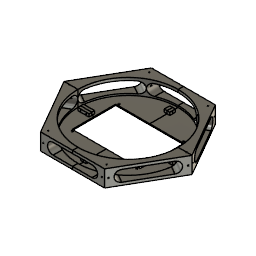
BoTech.StarClock.Top (Autodesk Fusion 360 design; units mm, degrees)
Autodesk Fusion 360 part; units mm, degrees
note: some values were not read from the file. Chosen so that the rebuilt part matches the saved one: which bodies a step acts on. Set by a fixed rule: which sketch regions a step uses.
sketch "Skizze1" plane through (0, 0, 0) normal (0, 0, 1) x (1, 0, 0)
  line L0 (-61, 39) -> (61, 39)
  line L1 (61, 39) -> (61, -39)
  line L2 (61, -39) -> (-61, -39)
  line L3 (-61, -39) -> (-61, 39)
  line L4 (0, 0) -> (0, 39)
  line L5 (61, 44.5) -> (61, -44.5)
  line L6 (61, -39) -> (55, -39)
  line L7 (55, -39) -> (55, -44.5)
  line L8 (55, -44.5) -> (61, -44.5)
  line L9 (61, -44.5) -> (61, -39)
  line L10 (-61, -39) -> (-55, -39)
  line L11 (-55, -39) -> (-55, -44.5)
  line L12 (-55, -44.5) -> (-61, -44.5)
  line L13 (-61, -44.5) -> (-61, -39)
  line L14 (-61, 39) -> (-55, 39)
  line L15 (-55, 39) -> (-55, 44.5)
  line L16 (-55, 44.5) -> (-61, 44.5)
  line L17 (-61, 44.5) -> (-61, 39)
  line L18 (61, 39) -> (55, 39)
  line L19 (55, 39) -> (55, 44.5)
  line L20 (55, 44.5) -> (61, 44.5)
  line L21 (61, 44.5) -> (61, 39)
  circle A0 centre (58, 42) radius 1.5
  circle A1 centre (-58, 42) radius 1.5
  circle A2 centre (-58, -42) radius 1.5
  line L22 (58, 42) -> (58, -42)
  circle A3 centre (58, -42) radius 1.5
  line L23 (-70, 50) -> (70, 50)
  line L24 (70, 50) -> (70, -50)
  line L25 (70, -50) -> (-70, -50)
  line L26 (-70, -50) -> (-70, 50)
  line L27 (115, 0) -> (57.5, 99.5929)
  line L28 (57.5, 99.5929) -> (-57.5, 99.5929)
  line L29 (-57.5, 99.5929) -> (-115, 0)
  line L30 (-115, 0) -> (-57.5, -99.5929)
  line L31 (-57.5, -99.5929) -> (57.5, -99.5929)
  line L32 (57.5, -99.5929) -> (115, 0)
  circle A4 centre (0, 0) radius 90
  line L33 (-57.5, 99.5929) -> (57.5, -99.5929)
  line L34 (57.5, 99.5929) -> (-57.5, -99.5929)
  line L35 (-115, 0) -> (115, 0)
  circle A5 centre (-105, 0) radius 1
  line L36 (-57.5, 99.5929) -> (-52.5, 90.9327)
  circle A6 centre (-52.5, 90.9327) radius 1
  line L37 (57.5, 99.5929) -> (52.5, 90.9327)
  circle A7 centre (52.5, 90.9327) radius 1
  line L38 (115, 0) -> (105, 0)
  circle A8 centre (105, 0) radius 1
  line L39 (57.5, -99.5929) -> (52.5, -90.9327)
  circle A9 centre (52.5, -90.9327) radius 1
  line L40 (-57.5, -99.5929) -> (-52.5, -90.9327)
  circle A10 centre (-52.5, -90.9327) radius 1
  line L41 (-0.0002, 220) -> (-190.5257, 109.9998)
  line L42 (-190.5257, 109.9998) -> (-190.5255, -110.0002)
  line L43 (-190.5255, -110.0002) -> (0.0002, -220)
  line L44 (0.0002, -220) -> (190.5257, -109.9998)
  line L45 (190.5257, -109.9998) -> (190.5255, 110.0002)
  line L46 (190.5255, 110.0002) -> (-0.0002, 220)
  line L47 (-0.0002, 220) -> (-57.5, 99.5929)
  line L48 (-0.0002, 220) -> (57.5, 99.5929)
  line L49 (57.5, 99.5929) -> (190.5255, 110.0002)
  line L50 (190.5255, 110.0002) -> (127.0171, 0.0001)
  line L51 (127.0171, 0.0001) -> (190.5257, -109.9998)
  line L52 (57.5, -99.5929) -> (190.5257, -109.9998)
  line L53 (57.5, -99.5929) -> (0.0002, -220)
  line L54 (-57.5, -99.5929) -> (0.0002, -220)
  line L55 (-57.5, -99.5929) -> (-190.5255, -110.0002)
  line L56 (-190.5255, -110.0002) -> (-115, 0)
  line L57 (-115, 0) -> (-190.5257, 109.9998)
  line L58 (-57.5, 99.5929) -> (-190.5257, 109.9998)
  line L59 (57.5, 99.5929) -> (0, 99.5929)
  dimension "d1" = 122
  dimension "d2" = 78
  dimension "d3" = 39
  dimension "d4" = 89
  dimension "d5" = 6
  dimension "d7" = 5.5
  dimension "d8" = 6
  dimension "d9" = 5.5
  dimension "d10" = 6
  dimension "d11" = 5.5
  dimension "d12" = 6
  dimension "d13" = 5.5
  dimension "d14" = 3
  dimension "d17" = 3
  dimension "d19" = 3
  dimension "d22" = 84
  dimension "d23" = 3
  dimension "d24" = 140
  dimension "d25" = 100
  dimension "d26" = 115
  dimension "d27" = 180
  dimension "d28" = 2
  dimension "d29" = 10
  dimension "d30" = 2
  dimension "d31" = 10
  dimension "d32" = 2
  dimension "d33" = 10
  dimension "d34" = 2
  dimension "d35" = 10
  dimension "d36" = 2
  dimension "d37" = 10
  dimension "d38" = 2
  dimension "d43" = 220
  dimension "d44" = 57.5
  constraint horizontal L0
  constraint vertical L1
  constraint horizontal L2
  constraint vertical L3
  constraint coincident L4.start A4.centre
  constraint perpendicular L2 L4
  constraint perpendicular L2 L5
  constraint coincident L2 L6.end
  constraint vertical L7
  constraint horizontal L8
  constraint vertical L9
  constraint horizontal L10
  constraint vertical L11
  constraint horizontal L12
  constraint vertical L13
  constraint horizontal L14
  constraint vertical L15
  constraint horizontal L16
  constraint vertical L17
  constraint horizontal L18
  constraint vertical L19
  constraint horizontal L20
  constraint vertical L21
  constraint perpendicular L0 L22
  constraint coincident A0.centre L22.start
  constraint coincident L22.end A3.centre
  constraint horizontal L23
  constraint vertical L24
  constraint horizontal L25
  constraint vertical L26
  constraint horizontal L35
  constraint coincident L35 A5.centre
  constraint coincident L33 L36.end
  constraint coincident L36.end A6.centre
  constraint coincident L34 L37.end
  constraint coincident L37.end A7.centre
  constraint coincident L35 L38.end
  constraint coincident L38.end A8.centre
  constraint coincident L33 L39.end
  constraint coincident L39.end A9.centre
  constraint coincident L34 L40.end
  constraint coincident L40.end A10.centre
  constraint perpendicular L46 L50
  constraint perpendicular L44 L51
  constraint parallel L28 L59
  measures "d1" distance of L0.start L0.end
  measures "d2" distance of L0.start L2.end
  measures "d3" distance of L4.start L4.end
  measures "d4" distance of L5.start L5.end
  measures "d5" distance of L1.end L6.end
  measures "d7" distance of L1.end L5.end
  measures "d8" distance of L2.end L10.end
  measures "d9" distance of L2.end L12.end
  measures "d10" distance of L0.start L14.end
  measures "d11" distance of L0.start L16.end
  measures "d12" distance of L0.end L18.end
  measures "d13" distance of L0.end L5.start
  measures "d14" diameter of A0
  measures "d17" diameter of A1
  measures "d19" diameter of A2
  measures "d22" distance of A0.centre L22.end
  measures "d23" diameter of A3
  measures "d24" distance of L23.start L23.end
  measures "d25" distance of L23.start L25.end
  measures "d26" distance of L27.start L4.start
  measures "d27" diameter of A4
  measures "d28" diameter of A5
  measures "d29" distance of L28.end L36.end
  measures "d30" diameter of A6
  measures "d31" distance of L27.end L37.end L4.start
  measures "d32" diameter of A7 L4.start
  measures "d33" distance of L27.start L38.end
  measures "d34" diameter of A8
  measures "d35" distance of L31.end L39.end
  measures "d36" diameter of A9
  measures "d37" distance of L30.end L40.end
  measures "d38" diameter of A10
  measures "d43" distance of L41.start L4.start
  measures "d44" distance of L27.end L59.end L4.start
extrude "Extrusion1" add sketch "Skizze1" along normal blind 30 contours L29 A4 L33 L35 A5 L36 A6 | L30 A4 L34 L35 A5 L40 A10 | L28 A4 L33 L34 L36 A6 L37 A7 L59 | L31 A4 L33 L34 L39 A9 L40 A10 | L27 A4 L34 L35 L37 A7 L38 A8 | L32 A4 L33 L35 L38 A8 L39 A9 makes body 1
extrude "Extrusion2" add sketch "Skizze1" along normal blind 2 contours L0 L14 L15 L16 L17 | L0 L3 L15 L16 L17 L23 L26 L33 L35 | L2 L3 L11 L12 L13 L25 L26 L34 L35 | L0 L23 L33 L34 | L2 L10 L11 L12 L13 | L23 L26 A4 L33 L35 | L25 L26 A4 L34 L35 | L23 A4 L33 L34 | L2 L25 L33 L34 | L1 L2 L5 L7 L8 L9 L24 L25 L33 L35 | L0 L1 L5 L19 L20 L21 L23 L24 L34 L35 | L23 L24 A4 L34 L35 | L25 A4 L33 L34 | L35 A5 | L35 A5 | L2 L5 L6 L7 L8 L9 | L24 L25 A4 L33 L35 | L0 L5 L18 L19 L20 L21 | L33 L36 A6 | L33 L36 A6 | L34 L40 A10 | L34 L40 A10 | L34 L37 A7 | L34 L37 A7 | L33 L39 A9 | L33 L39 A9 | L35 L38 A8 | L35 L38 A8 bodies 1
sketch "Skizze2" plane through (0, -99.5929, 0) normal (0, -1, 0) x (1, 0, 0)
  line L0 (-57.5, 0) -> (57.5, 0)
  line L1 (57.5, 0) -> (57.5, 30)
  line L2 (57.5, 30) -> (-57.5, 30)
  line L3 (-57.5, 30) -> (-57.5, 0)
  line L4 (57.5, 30) -> (57.5, 0)
  line L5 (-57.5, 30) -> (57.5, 30)
  circle A0 centre (-52.5, 15) radius 2.5
  circle A1 centre (52.5, 15) radius 3.5
  circle A2 centre (-52.5, 15) radius 3.5
  line L6 (-57.5, 0) -> (-57.5, 30)
  circle A3 centre (52.5, 15) radius 1
  line L7 (47.5, 0) -> (47.5, 30)
  circle A4 centre (-52.5, 15) radius 1
  line L8 (57.5, 0) -> (-57.5, 0)
  line L9 (-47.5, 30) -> (-47.5, 0)
  circle A5 centre (52.5, 15) radius 2.5
  line L10 (-35, 25) -> (35, 25)
  line L11 (35, 25) -> (35, 5)
  line L12 (35, 5) -> (-35, 5)
  arc A6 (-35, 25) -> (-35, 5) centre (-35, 15) ccw
  arc A7 (35, 5) -> (35, 25) centre (35, 15) ccw
  point P0 (-57.5, 15)
  dimension "d45" = 115
  dimension "d46" = 30
  dimension "d47" = 2
  dimension "d48" = 5
  dimension "d49" = 2
  dimension "d50" = 5
  constraint horizontal L8
  constraint vertical L6
  constraint horizontal L5
  constraint vertical L4
  constraint concentric A3 A5
  constraint concentric A0 A4
  constraint coincident L9.start L5
  constraint coincident L9.end L8
  constraint perpendicular L8 L9
  constraint coincident L7.start L8
  constraint coincident L7.end L5
  constraint perpendicular L5 L7
  constraint concentric A0 A2
  constraint concentric A1 A3
  constraint parallel L5 L10
  constraint perpendicular L8 L11
  constraint perpendicular L11 L12
  constraint tangent L10 A6
  constraint tangent L12 A7
  measures "d45" distance of L0.end L0.start
  measures "d46" distance of L0.end L1.end
  measures "d47" diameter of A3
  measures "d48" diameter of A5
  measures "d49" diameter of A4
  measures "d50" diameter of A0
sketch "Skizze3" plane through (86.25, -49.7965, 0) normal (0.866025, -0.5, 0) x (0.5, 0.866025, 0)
  line L0 (-57.5, 0) -> (57.5, 0)
  line L1 (57.5, 0) -> (57.5, 30)
  line L2 (57.5, 30) -> (-57.5, 30)
  line L3 (-57.5, 30) -> (-57.5, 0)
  line L4 (35, 5) -> (-35, 5)
  arc A0 (-35, 25) -> (-35, 5) centre (-35, 15) ccw
  circle A1 centre (-52.5, 15) radius 3.5
  circle A2 centre (52.5, 15) radius 1
  line L5 (57.5, 30) -> (57.5, 0)
  line L6 (35, 25) -> (35, 5)
  line L7 (-47.5, 30) -> (-47.5, 0)
  circle A3 centre (52.5, 15) radius 2.5
  line L8 (57.5, 0) -> (57.5, 30)
  circle A4 centre (-52.5, 15) radius 2.5
  line L9 (-57.5, 0) -> (57.5, 0)
  circle A5 centre (52.5, 15) radius 3.5
  arc A6 (35, 5) -> (35, 25) centre (35, 15) ccw
  line L10 (57.5, 0) -> (-57.5, 0)
  line L11 (-57.5, 30) -> (57.5, 30)
  line L12 (-57.5, 0) -> (-57.5, 30)
  circle A7 centre (-52.5, 15) radius 1
  line L13 (-35, 25) -> (35, 25)
  line L14 (-57.5, 30) -> (-57.5, 0)
  line L15 (47.5, 0) -> (47.5, 30)
  line L16 (57.5, 30) -> (-57.5, 30)
  point P0 (-57.5, 15)
  dimension "d53" = 115
  dimension "d54" = 30
  dimension "d55" = 2
  dimension "d56" = 5
  dimension "d57" = 2
  dimension "d58" = 5
  constraint horizontal L10
  constraint vertical L12
  constraint horizontal L11
  constraint vertical L5
  constraint concentric A2 A3
  constraint concentric A4 A7
  constraint coincident L7.start L11
  constraint coincident L7.end L10
  constraint perpendicular L7 L10
  constraint coincident L15.start L10
  constraint coincident L15.end L11
  constraint perpendicular L11 L15
  constraint concentric A1 A4
  constraint concentric A2 A5
  constraint parallel L11 L13
  constraint perpendicular L6 L10
  constraint perpendicular L4 L6
  constraint tangent A0 L13
  constraint tangent L4 A6
  measures "d53" distance of L0.start L0.end
  measures "d54" distance of L1.end L0.end
  measures "d55" diameter of A2
  measures "d56" diameter of A3
  measures "d57" diameter of A7
  measures "d58" diameter of A4
sketch "Skizze4" plane through (86.25, 49.7965, 0) normal (0.866025, 0.5, 0) x (-0.5, 0.866025, 0)
  line L0 (-57.5, 0) -> (57.5, 0)
  line L1 (57.5, 0) -> (57.5, 30)
  line L2 (57.5, 30) -> (-57.5, 30)
  line L3 (-57.5, 30) -> (-57.5, 0)
  line L4 (35, 5) -> (-35, 5)
  arc A0 (-35, 25) -> (-35, 5) centre (-35, 15) ccw
  circle A1 centre (-52.5, 15) radius 3.5
  circle A2 centre (52.5, 15) radius 1
  line L5 (57.5, 30) -> (57.5, 0)
  line L6 (35, 25) -> (35, 5)
  line L7 (-47.5, 30) -> (-47.5, 0)
  circle A3 centre (52.5, 15) radius 2.5
  line L8 (57.5, 0) -> (57.5, 30)
  circle A4 centre (-52.5, 15) radius 2.5
  line L9 (-57.5, 0) -> (57.5, 0)
  circle A5 centre (52.5, 15) radius 3.5
  arc A6 (35, 5) -> (35, 25) centre (35, 15) ccw
  line L10 (57.5, 0) -> (-57.5, 0)
  line L11 (-57.5, 30) -> (57.5, 30)
  line L12 (-57.5, 0) -> (-57.5, 30)
  circle A7 centre (-52.5, 15) radius 1
  line L13 (-35, 25) -> (35, 25)
  line L14 (-57.5, 30) -> (-57.5, 0)
  line L15 (47.5, 0) -> (47.5, 30)
  line L16 (57.5, 30) -> (-57.5, 30)
  point P0 (-57.5, 15)
  dimension "d59" = 115
  dimension "d60" = 30
  dimension "d61" = 2
  dimension "d62" = 5
  dimension "d63" = 2
  dimension "d64" = 5
  constraint horizontal L10
  constraint vertical L12
  constraint horizontal L11
  constraint vertical L5
  constraint concentric A2 A3
  constraint concentric A4 A7
  constraint coincident L7.start L11
  constraint coincident L7.end L10
  constraint perpendicular L7 L10
  constraint coincident L15.start L10
  constraint coincident L15.end L11
  constraint perpendicular L11 L15
  constraint concentric A1 A4
  constraint concentric A2 A5
  constraint parallel L11 L13
  constraint perpendicular L6 L10
  constraint perpendicular L4 L6
  constraint tangent A0 L13
  constraint tangent L4 A6
  measures "d59" distance of L0.start L0.end
  measures "d60" distance of L1.end L0.end
  measures "d61" diameter of A2
  measures "d62" diameter of A3
  measures "d63" diameter of A7
  measures "d64" diameter of A4
sketch "Skizze5" plane through (0, 99.5929, 0) normal (0, 1, 0) x (-1, 0, 0)
  line L0 (-57.5, 0) -> (57.5, 0)
  line L1 (57.5, 0) -> (57.5, 30)
  line L2 (57.5, 30) -> (-57.5, 30)
  line L3 (-57.5, 30) -> (-57.5, 0)
  line L4 (35, 5) -> (-35, 5)
  arc A0 (-35, 25) -> (-35, 5) centre (-35, 15) ccw
  circle A1 centre (-52.5, 15) radius 3.5
  circle A2 centre (52.5, 15) radius 1
  line L5 (57.5, 30) -> (57.5, 0)
  line L6 (35, 25) -> (35, 5)
  line L7 (-47.5, 30) -> (-47.5, 0)
  circle A3 centre (52.5, 15) radius 2.5
  line L8 (57.5, 0) -> (57.5, 30)
  circle A4 centre (-52.5, 15) radius 2.5
  line L9 (-57.5, 0) -> (57.5, 0)
  circle A5 centre (52.5, 15) radius 3.5
  arc A6 (35, 5) -> (35, 25) centre (35, 15) ccw
  line L10 (57.5, 0) -> (-57.5, 0)
  line L11 (-57.5, 30) -> (57.5, 30)
  line L12 (-57.5, 0) -> (-57.5, 30)
  circle A7 centre (-52.5, 15) radius 1
  line L13 (-35, 25) -> (35, 25)
  line L14 (-57.5, 30) -> (-57.5, 0)
  line L15 (47.5, 0) -> (47.5, 30)
  line L16 (57.5, 30) -> (-57.5, 30)
  point P0 (-57.5, 15)
  dimension "d65" = 115
  dimension "d66" = 30
  dimension "d67" = 2
  dimension "d68" = 5
  dimension "d69" = 2
  dimension "d70" = 5
  constraint horizontal L10
  constraint vertical L12
  constraint horizontal L11
  constraint vertical L5
  constraint concentric A2 A3
  constraint concentric A4 A7
  constraint coincident L7.start L11
  constraint coincident L7.end L10
  constraint perpendicular L7 L10
  constraint coincident L15.start L10
  constraint coincident L15.end L11
  constraint perpendicular L11 L15
  constraint concentric A1 A4
  constraint concentric A2 A5
  constraint parallel L11 L13
  constraint perpendicular L6 L10
  constraint perpendicular L4 L6
  constraint tangent A0 L13
  constraint tangent L4 A6
  measures "d65" distance of L0.start L0.end
  measures "d66" distance of L1.end L0.end
  measures "d67" diameter of A2
  measures "d68" diameter of A3
  measures "d69" diameter of A7
  measures "d70" diameter of A4
sketch "Skizze6" plane through (-86.25, 49.7965, 0) normal (-0.866025, 0.5, 0) x (-0.5, -0.866025, 0)
  line L0 (-57.5, 0) -> (57.5, 0)
  line L1 (57.5, 0) -> (57.5, 30)
  line L2 (57.5, 30) -> (-57.5, 30)
  line L3 (-57.5, 30) -> (-57.5, 0)
  line L4 (35, 5) -> (-35, 5)
  arc A0 (-35, 25) -> (-35, 5) centre (-35, 15) ccw
  circle A1 centre (-52.5, 15) radius 3.5
  circle A2 centre (52.5, 15) radius 1
  line L5 (57.5, 30) -> (57.5, 0)
  line L6 (35, 25) -> (35, 5)
  line L7 (-47.5, 30) -> (-47.5, 0)
  circle A3 centre (52.5, 15) radius 2.5
  line L8 (57.5, 0) -> (57.5, 30)
  circle A4 centre (-52.5, 15) radius 2.5
  line L9 (-57.5, 0) -> (57.5, 0)
  circle A5 centre (52.5, 15) radius 3.5
  arc A6 (35, 5) -> (35, 25) centre (35, 15) ccw
  line L10 (57.5, 0) -> (-57.5, 0)
  line L11 (-57.5, 30) -> (57.5, 30)
  line L12 (-57.5, 0) -> (-57.5, 30)
  circle A7 centre (-52.5, 15) radius 1
  line L13 (-35, 25) -> (35, 25)
  line L14 (-57.5, 30) -> (-57.5, 0)
  line L15 (47.5, 0) -> (47.5, 30)
  line L16 (57.5, 30) -> (-57.5, 30)
  point P0 (-57.5, 15)
  dimension "d71" = 115
  dimension "d72" = 30
  dimension "d73" = 2
  dimension "d74" = 5
  dimension "d75" = 2
  dimension "d76" = 5
  constraint horizontal L10
  constraint vertical L12
  constraint horizontal L11
  constraint vertical L5
  constraint concentric A2 A3
  constraint concentric A4 A7
  constraint coincident L7.start L11
  constraint coincident L7.end L10
  constraint perpendicular L7 L10
  constraint coincident L15.start L10
  constraint coincident L15.end L11
  constraint perpendicular L11 L15
  constraint concentric A1 A4
  constraint concentric A2 A5
  constraint parallel L11 L13
  constraint perpendicular L6 L10
  constraint perpendicular L4 L6
  constraint tangent A0 L13
  constraint tangent L4 A6
  measures "d71" distance of L0.start L0.end
  measures "d72" distance of L1.end L0.end
  measures "d73" diameter of A2
  measures "d74" diameter of A3
  measures "d75" diameter of A7
  measures "d76" diameter of A4
sketch "Skizze7" plane through (-86.25, -49.7965, 0) normal (-0.866025, -0.5, 0) x (0.5, -0.866025, 0)
  line L0 (-57.5, 0) -> (57.5, 0)
  line L1 (57.5, 0) -> (57.5, 30)
  line L2 (57.5, 30) -> (-57.5, 30)
  line L3 (-57.5, 30) -> (-57.5, 0)
  line L4 (35, 5) -> (-35, 5)
  arc A0 (-35, 25) -> (-35, 5) centre (-35, 15) ccw
  circle A1 centre (-52.5, 15) radius 3.5
  circle A2 centre (52.5, 15) radius 1
  line L5 (57.5, 30) -> (57.5, 0)
  line L6 (35, 25) -> (35, 5)
  line L7 (-47.5, 30) -> (-47.5, 0)
  circle A3 centre (52.5, 15) radius 2.5
  line L8 (57.5, 0) -> (57.5, 30)
  circle A4 centre (-52.5, 15) radius 2.5
  line L9 (-57.5, 0) -> (57.5, 0)
  circle A5 centre (52.5, 15) radius 3.5
  arc A6 (35, 5) -> (35, 25) centre (35, 15) ccw
  line L10 (57.5, 0) -> (-57.5, 0)
  line L11 (-57.5, 30) -> (57.5, 30)
  line L12 (-57.5, 0) -> (-57.5, 30)
  circle A7 centre (-52.5, 15) radius 1
  line L13 (-35, 25) -> (35, 25)
  line L14 (-57.5, 30) -> (-57.5, 0)
  line L15 (47.5, 0) -> (47.5, 30)
  line L16 (57.5, 30) -> (-57.5, 30)
  point P0 (-57.5, 15)
  dimension "d77" = 115
  dimension "d78" = 30
  dimension "d79" = 2
  dimension "d80" = 5
  dimension "d81" = 2
  dimension "d82" = 5
  constraint horizontal L10
  constraint vertical L12
  constraint horizontal L11
  constraint vertical L5
  constraint concentric A2 A3
  constraint concentric A4 A7
  constraint coincident L7.start L11
  constraint coincident L7.end L10
  constraint perpendicular L7 L10
  constraint coincident L15.start L10
  constraint coincident L15.end L11
  constraint perpendicular L11 L15
  constraint concentric A1 A4
  constraint concentric A2 A5
  constraint parallel L11 L13
  constraint perpendicular L6 L10
  constraint perpendicular L4 L6
  constraint tangent A0 L13
  constraint tangent L4 A6
  measures "d77" distance of L0.start L0.end
  measures "d78" distance of L1.end L0.end
  measures "d79" diameter of A2
  measures "d80" diameter of A3
  measures "d81" diameter of A7
  measures "d82" diameter of A4
extrude "Extrusion3" cut sketch "Skizze2" against normal blind 28 contours A3 | A4 | L10 L11 L12 A6 | L11 A7 bodies 1
extrude "Extrusion4" cut sketch "Skizze3" against normal blind 28 contours L4 A0 L6 L13 | L6 A6 | A2 | A7 bodies 1
extrude "Extrusion5" cut sketch "Skizze4" against normal blind 28 contours L4 A0 L6 L13 | L6 A6 | A2 | A7 bodies 1
extrude "Extrusion6" cut sketch "Skizze5" against normal blind 28 contours L4 A0 L6 L13 | L6 A6 | A2 | A7 bodies 1
extrude "Extrusion7" cut sketch "Skizze6" against normal blind 28 contours L4 A0 L6 L13 | L6 A6 | A2 | A7 bodies 1
extrude "Extrusion8" cut sketch "Skizze7" against normal blind 28 contours L4 A0 L6 L13 | L6 A6 | A2 | A7 bodies 1
sketch "Skizze8" plane through (0, 0, 2) normal (0, 0, 1) x (-1, 0, 0)
  circle A0 centre (-58, -42) radius 1.5
  circle A1 centre (-58, 42) radius 1.5
  line L0 (-61, -39) -> (-61, 39)
  line L1 (-61, 39) -> (61, 39)
  line L2 (61, 39) -> (61, -39)
  line L3 (61, -39) -> (-61, -39)
  circle A2 centre (58, 42) radius 1.5
  circle A3 centre (58, -42) radius 1.5
  circle A4 centre (0, 0) radius 90
  line L4 (65, 5) -> (85, 5)
  line L5 (85, 5) -> (85, -5)
  line L6 (85, -5) -> (65, -5)
  line L7 (65, -5) -> (65, 5)
  line L8 (0, -20) -> (0, 10)
  line L9 (-85, -5) -> (-65, -5)
  line L10 (-65, -5) -> (-65, 5)
  line L11 (-85, 5) -> (-85, -5)
  line L12 (-65, 5) -> (-85, 5)
  line L13 (5, 80) -> (-5, 80)
  line L14 (-5, 80) -> (-5, 70)
  line L15 (-5, 70) -> (5, 70)
  line L16 (5, 70) -> (5, 80)
  line L17 (15, 0) -> (-20, 0)
  line L18 (5, -80) -> (-5, -80)
  line L19 (-5, -80) -> (-5, -70)
  line L20 (5, -70) -> (5, -80)
  line L21 (-5, -70) -> (5, -70)
  dimension "d101" = 10
  dimension "d102" = 10
  constraint horizontal L4
  constraint vertical L5
  constraint horizontal L6
  constraint vertical L7
  constraint vertical L8
  constraint symmetric L4.start L8 L10.end
  constraint symmetric L4.end L8 L11.start
  constraint symmetric L5.end L8 L9.start
  constraint symmetric L6.end L8 L9.end
  constraint horizontal L13
  constraint vertical L14
  constraint horizontal L15
  constraint vertical L16
  constraint perpendicular L8 L17
  constraint symmetric L13.start L17 L18.start
  constraint symmetric L13.end L17 L18.end
  constraint symmetric L14.end L17 L19.end
  constraint symmetric L15.end L17 L20.start
  measures "d101" distance of L13.start L13.end
  measures "d102" distance of L13.start L15.end
extrude "Extrusion9" add sketch "Skizze8" along normal blind 5 contours L4 L5 L6 L7 | L9 L10 L11 L12 | L13 L14 L15 L16 | L18 L19 L20 L21 bodies 1
sketch "Skizze9" plane through (0, -5, 0) normal (0, -1, 0) x (1, 0, 0)
  line L0 (-85, 2) -> (-65, 2)
  line L1 (-65, 2) -> (-65, 7)
  line L2 (-65, 7) -> (-85, 7)
  line L3 (-85, 7) -> (-85, 2)
  line L4 (-85, 7) -> (-65, 7)
  line L5 (-65, 7) -> (-65, 2)
  line L6 (-65, 2) -> (-85, 2)
  line L7 (-85, 2) -> (-85, 7)
  line L8 (-85, 4.5) -> (-80, 4.5)
  circle A0 centre (-80, 4.5) radius 1
  line L9 (-65, 4.5) -> (-70, 4.5)
  circle A1 centre (-70, 4.5) radius 1
  line L10 (0, 0) -> (0, 25)
  line L11 (65, 2) -> (65, 7)
  line L12 (85, 2) -> (65, 2)
  line L13 (65, 2) -> (85, 2)
  line L14 (85, 7) -> (85, 2)
  line L15 (65, 7) -> (85, 7)
  line L16 (85, 7) -> (65, 7)
  line L17 (65, 4.5) -> (70, 4.5)
  circle A2 centre (70, 4.5) radius 1
  line L18 (65, 7) -> (65, 2)
  line L19 (85, 4.5) -> (80, 4.5)
  circle A3 centre (80, 4.5) radius 1
  line L20 (85, 2) -> (85, 7)
  dimension "d95" = 2
  dimension "d96" = 5
  dimension "d97" = 2
  dimension "d98" = 5
  constraint horizontal L4
  constraint vertical L5
  constraint horizontal L6
  constraint vertical L7
  constraint coincident L0.end L1.start
  constraint coincident L2.end L3.start
  constraint midpoint L7 L8.start
  constraint perpendicular L5 L8
  constraint coincident L8.end A0.centre
  constraint midpoint L5 L9.start
  constraint perpendicular L5 L9
  constraint coincident L9.end A1.centre
  constraint coincident L10.start origin
  constraint vertical L10
  constraint symmetric L0.start L10 L12.start
  constraint symmetric L0.end L10 L11.start
  constraint symmetric L1.end L10 L11.end
  constraint symmetric L2.end L10 L14.start
  constraint symmetric L8.start L10 L19.start
  constraint symmetric L8.end L10 L19.end
  constraint symmetric A0 L10 A3
  constraint symmetric L9.start L10 L17.start
  constraint symmetric L9.end L10 L17.end
  constraint symmetric A1 L10 A2
  measures "d95" diameter of A0
  measures "d96" distance of L9.start L9.end
  measures "d97" diameter of A1
  measures "d98" distance of L8.start L8.end
sketch "Skizze10" plane through (-5, 0, 0) normal (-1, 0, 0) x (0, -1, 0)
  line L0 (-80, 2) -> (-70, 2)
  line L1 (-70, 2) -> (-70, 7)
  line L2 (-70, 7) -> (-80, 7)
  line L3 (-80, 7) -> (-80, 2)
  line L4 (-80, 2) -> (-70, 2)
  line L5 (-70, 2) -> (-70, 7)
  line L6 (-70, 7) -> (-80, 7)
  line L7 (-80, 7) -> (-80, 2)
  circle A0 centre (-75, 4.5) radius 1
  line L8 (0, 0) -> (0, 11)
  circle A1 centre (75, 4.5) radius 1
  line L9 (80, 2) -> (70, 2)
  line L10 (70, 2) -> (70, 7)
  line L11 (80, 2) -> (70, 2)
  line L12 (70, 2) -> (70, 7)
  line L13 (80, 7) -> (80, 2)
  line L14 (70, 7) -> (80, 7)
  line L15 (80, 7) -> (80, 2)
  line L16 (70, 7) -> (80, 7)
  dimension "d103" = 2
  constraint horizontal L4
  constraint vertical L5
  constraint horizontal L6
  constraint vertical L7
  constraint coincident L1.end L2.start
  constraint coincident L0.start L3.end
  constraint coincident L8.start origin
  constraint vertical L8
  constraint symmetric L0.start L8 L9.start
  constraint symmetric L0.end L8 L9.end
  constraint symmetric L1.end L8 L10.end
  constraint symmetric L2.end L8 L13.start
  constraint symmetric A0 L8 A1
  measures "d103" diameter of A0
extrude "Extrusion11" cut sketch "Skizze10" against normal blind 10 contours A0 | A1 bodies 1
extrude "Extrusion10" cut sketch "Skizze9" against normal blind 10 contours A0 | A1 | A2 | A3 bodies 1
split "Teilen1" by curves path "Skizze1" along L35 bodies 1 makes body 2 at (18.8936, -80.6333, 0)
split "Teilen2" by curves path "Skizze1" along L4 bodies 2 1 makes body 3 at (18.954, 60.5233, 0) makes body 4 at (18.954, -60.5233, 0)
copy_body "Körper->Berechn3" bodies 1 removing the originals makes body 5 in component "BoTech.StarClock.Top.A"
copy_body "Körper->Berechn4" bodies 2 removing the originals makes body 6 in component "BoTech.StarClock.Top.B"
copy_body "Körper->Berechn5" bodies 3 removing the originals makes body 7 in component "BoTech.StarClock.Top.C"
copy_body "Körper->Berechn6" bodies 4 removing the originals makes body 8 in component "BoTech.StarClock.Top.D"
component "BoTech.StarClock.Top.A" placed x (1, 0, 0) y (0, 1, 0) z (0, 0, 1) at (0, 0, 0)
component "BoTech.StarClock.Top.B" placed x (1, 0, 0) y (0, 1, 0) z (0, 0, 1) at (0, 0, 0)
component "BoTech.StarClock.Top.C" placed x (1, 0, 0) y (0, 1, 0) z (0, 0, 1) at (0, 0, 0)
component "BoTech.StarClock.Top.D" placed x (1, 0, 0) y (0, 1, 0) z (0, 0, 1) at (0, 0, 0)
